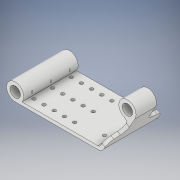
# Autodesk Inventor part: Turret Sensor Mount
Saved by Autodesk Inventor 2019.4 (Build 234330000, 330)
## iProperties
Created: 2020-01-25
Part Number: Turret Sensor Mount
Material: ABS Plastic
Document SubType Name: Modeling
Designer: admin
Density: 1.95534 g/cm^3
Appearance: Smooth - White
Mass: 200 g
Surface Area: 460.142 cm^2
Volume: 112.905 cm^3
Author: admin
Autodesk Inventor part; units mm, degrees
ref_plane "YZ Plane" through (0, 0, 0) normal (1, 0, 0) x (0, 1, 0)
ref_plane "XZ Plane" through (0, 0, 0) normal (0, 1, 0) x (-1, 0, 0)
ref_plane "XY Plane" through (0, 0, 0) normal (0, 0, 1) x (1, 0, 0)
sketch "Sketch1" plane through (0, 0, 0) normal (0, 0, 1) x (1, 0, 0)
  circle A0 centre (0, 0) radius 7.7
  circle A1 centre (0, 0) radius 12.7
  line L0 (0, 0) -> (140.2808, 0) construction
  line L1 (140.2808, 0) -> (140.2808, 34.9) construction
  circle A2 centre (140.2808, 34.9) radius 7.7
  circle A3 centre (140.2808, 34.9) radius 12.7
  line L2 (0, 0) -> (140.2808, 34.9) construction
  dimension "d0" = 15.4
  dimension "d3" = 5
  dimension "d13" = 15.4
  dimension "d14" = 5
  dimension "d15" = 34.9
  dimension "d16" = 144.557
  constraints: 6 end point, 4 centre point, 4 coincident, 1 horizontal, 1 vertical
  measures "d0" diameter of A0
  measures "d3" radial gap between concentric circles of A0 A1
  measures "d13" diameter of A2
  measures "d14" radial gap between concentric circles of A3 A2
  measures "d15" distance of L0.end L1.end
  measures "d16" distance of L0.start L2.end
extrude "Extrusion1" add sketch "Sketch1" along normal blind 80
sketch "Sketch3" plane through (0, 0, 80) normal (0, 0, 1) x (1, 0, 0)
  circle A0 centre (0, 0) radius 12.7 projected
  line L0 (124.5769, -7.7) -> (141.8995, 22.3036)
  circle A1 centre (140.2808, 34.9) radius 12.7 projected
  line L1 (0, -12.7) -> (127.4637, -12.7)
  line L2 (127.4637, -12.7) -> (151.2794, 28.55)
  line L3 (124.5769, -7.7) -> (10.0995, -7.7)
  point P0 (0, 12.7)
  dimension "d18" = 5
  dimension "d24" = 5
  dimension "d25" = 120
  constraints: 8 end point, 5 point on circle, 2 horizontal, 2 tangent, 1 parallel
  measures "d18" distance between parallel lines of L2 L0
  measures "d24" distance between parallel lines of L1 L3
  measures "d25" angle of L3 L0
extrude "Extrusion3" add sketch "Sketch3" against normal up to surface (80 mm away) contours A0 L3 L0 A1 L2 L1
fillet "Fillet2" radius 5 3 edges at (141.8995, 22.3036, 40) (124.5769, -7.7, 40) (0, -12.7, 40)
fillet "Fillet3" radius 10 1 edges at (127.4637, -12.7, 40)
sketch "Sketch4" plane through (151.2794, 28.55, 80) normal (0.8660254, -0.5, 0) x (0, 0, -1)
  line L0 (80, -41.8579) -> (80, -17.4929) projected
  line L1 (80, -29.6754) -> (55, -24.6754)
  line L2 (55, -24.6754) -> (55, 12.7)
  line L3 (55, 12.7) -> (25, 12.7)
  line L4 (80, 12.7) -> (0, 12.7) projected
  line L5 (25, 12.7) -> (25, -24.6754)
  line L6 (25, -24.6754) -> (0, -29.6754)
  line L7 (0, -41.8579) -> (0, 0) projected
  line L8 (80, -29.6754) -> (80, 12.7)
  line L9 (80, 12.7) -> (55, 12.7)
  line L10 (25, 12.7) -> (0, 12.7)
  line L11 (0, -29.6754) -> (0, 12.7)
  point P0 (80, -100.3647)
  point P1 (40, 12.7)
  dimension "d26" = 5
  dimension "d27" = 30
  dimension "d29" = 5
  constraints: 18 end point, 3 midpoint, 2 collinear, 2 parallel, 2 perpendicular, 2 point on line, 2 vertical
  measures "d26" vertical distance of L1.start L1.end
  measures "d27" distance between parallel lines of L5 L2
  measures "d29" vertical distance of L5.end L6.end
extrude "Extrusion4" cut sketch "Sketch4" against normal through all
fillet "Fillet4" radius 10 4 edges at (134.2766, 4.1004, 0) (136.7766, 8.4305, 25) (136.7766, 8.4305, 55) (134.2766, 4.1004, 80)
sketch "Sketch5" plane through (0, -12.7, 0) normal (0, -1, 0) x (1, 0, 0)
  circle A0 centre (113.6902, 17.851) radius 2.5
  circle A1 centre (113.6902, 62.149) radius 2.5
  line L0 (113.6902, 62.149) -> (113.6902, 17.851) construction
  line L1 (113.6902, 40) -> (121.6902, 40) construction
  line L2 (121.6902, 0) -> (121.6902, 80) projected
  point P0 (0, 0)
  dimension "d33" = 5
  dimension "d34" = 5
  dimension "d35" = 44.298
  dimension "d36" = 8
  constraints: 4 end point, 2 centre point, 2 midpoint, 2 perpendicular
  measures "d33" diameter of A0
  measures "d34" diameter of A1
  measures "d35" distance of L0.start L0.end
  measures "d36" distance between parallel lines of L2 L0
extrude "Extrusion5" cut sketch "Sketch5" against normal through all
sketch "Sketch6" plane through (0, -12.7, 0) normal (0, -1, 0) x (1, 0, 0)
  circle A0 centre (15, 12.5) radius 2.5
  circle A1 centre (15, 40) radius 2.5
  circle A2 centre (15, 67.5) radius 2.5
  line L0 (15, 12.5) -> (15, 67.5) construction
  line L1 (15, 40) -> (0, 40) construction
  line L2 (0, 0) -> (0, 80) construction
  circle A3 centre (30, 12.5) radius 2.5
  circle A4 centre (30, 40) radius 2.5
  circle A5 centre (30, 67.5) radius 2.5
  circle A6 centre (45, 12.5) radius 2.5
  circle A7 centre (45, 40) radius 2.5
  circle A8 centre (45, 67.5) radius 2.5
  circle A9 centre (60, 12.5) radius 2.5
  circle A10 centre (60, 40) radius 2.5
  circle A11 centre (60, 67.5) radius 2.5
  circle A12 centre (75, 12.5) radius 2.5
  circle A13 centre (75, 40) radius 2.5
  circle A14 centre (75, 67.5) radius 2.5
  dimension "d39" = 5
  dimension "d40" = 5
  dimension "d41" = 5
  dimension "d42" = 15
  dimension "d45" = 15
  dimension "d50" = 55
  constraints: 15 centre point, 4 end point, 2 midpoint, 1 horizontal, 1 perpendicular, 1 vertical, 24 other
  measures "d39" diameter of A0
  measures "d40" diameter of A1
  measures "d41" diameter of A2
  measures "d42" distance of L1.start L1.end
  measures "d45" distance of L0.start A3.centre
  measures "d50" distance of L0.start L0.end
extrude "Extrusion6" cut sketch "Sketch6" against normal through all
equation "\"d29\" = d26"
body "Solid1"
